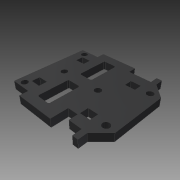
# Autodesk Inventor part: x_motor_middle
Saved by Autodesk Inventor 2014 (Build 180170000, 170)
## iProperties
Created: 2013-12-01
Part Number: x_motor_middle
Material: Generic
Document SubType Name: Modeling
Designer: buben
Density: 1 g/cm^3
Appearance: Anodized - Dark Gray
Author: buben
Subject: Laser Cutted
Autodesk Inventor part; units mm, degrees
ref_plane "YZ Plane" through (0, 0, 0) normal (1, 0, 0) x (0, 1, 0)
ref_plane "XZ Plane" through (0, 0, 0) normal (0, 1, 0) x (-1, 0, 0)
ref_plane "XY Plane" through (0, 0, 0) normal (0, 0, 1) x (1, 0, 0)
sketch "Sketch1" plane through (0, 0, 0) normal (0, 0, 1) x (1, 0, 0)
  line L0 (0, 68.5) -> (0, 6.5)
  line L1 (68, 68.5) -> (78, 58.5)
  line L2 (78, 58.5) -> (78, 16.5)
  line L3 (78, 16.5) -> (68, 6.5)
  line L4 (68, 0) -> (68, 6.5)
  line L5 (68, 68.5) -> (68, 75)
  circle A0 centre (71, 57.5) radius 2.75
  circle A1 centre (71, 17.5) radius 2.75
  line L6 (25, 67.5) -> (34, 67.5)
  line L7 (35, 66.5) -> (35, 43.5)
  line L8 (34, 42.5) -> (25, 42.5)
  line L9 (24, 43.5) -> (24, 66.5)
  line L10 (25, 32.5) -> (34, 32.5)
  line L11 (35, 31.5) -> (35, 8.5)
  line L12 (34, 7.5) -> (25, 7.5)
  line L13 (24, 8.5) -> (24, 31.5)
  arc A2 (25, 67.5) -> (24, 66.5) centre (25, 66.5) ccw
  arc A3 (35, 66.5) -> (34, 67.5) centre (34, 66.5) ccw
  arc A4 (34, 42.5) -> (35, 43.5) centre (34, 43.5) ccw
  arc A5 (24, 43.5) -> (25, 42.5) centre (25, 43.5) ccw
  arc A6 (25, 32.5) -> (24, 31.5) centre (25, 31.5) ccw
  arc A7 (24, 8.5) -> (25, 7.5) centre (25, 8.5) ccw
  arc A8 (34, 7.5) -> (35, 8.5) centre (34, 8.5) ccw
  arc A9 (35, 31.5) -> (34, 32.5) centre (34, 31.5) ccw
  line L14 (29.5, 67.5) -> (29.5, 7.5) construction
  circle A10 centre (6, 64.5) radius 5 construction
  circle A11 centre (6, 64.5) radius 2.75
  circle A12 centre (6, 10.5) radius 5 construction
  circle A13 centre (6, 10.5) radius 2.75
  line L15 (0, 64.5) -> (72, 64.5) construction
  line L16 (0, 10.5) -> (72, 10.5) construction
  line L17 (0, 6.5) -> (16, 6.5)
  line L18 (16, 6.5) -> (16, 0)
  line L19 (0, 68.5) -> (16, 68.5)
  line L20 (16, 68.5) -> (16, 75)
  line L21 (46, 75) -> (46, 68.5)
  line L22 (46, 68.5) -> (64, 68.5)
  line L23 (64, 68.5) -> (64, 75)
  line L24 (46, 0) -> (46, 6.5)
  line L25 (46, 6.5) -> (64, 6.5)
  line L26 (64, 6.5) -> (64, 0)
  line L27 (68, 75) -> (64, 75)
  line L28 (46, 75) -> (16, 75)
  line L29 (16, 0) -> (46, 0)
  line L30 (64, 0) -> (68, 0)
  line L31 (8, 60.5) -> (16, 60.5)
  line L32 (16, 60.5) -> (16, 54)
  line L33 (16, 54) -> (8, 54)
  line L34 (8, 54) -> (8, 60.5)
  line L35 (8, 21) -> (16, 21)
  line L36 (16, 21) -> (16, 14.5)
  line L37 (16, 14.5) -> (8, 14.5)
  line L38 (8, 14.5) -> (8, 21)
  line L39 (54, 21) -> (62, 21)
  line L40 (62, 21) -> (62, 14.5)
  line L41 (62, 14.5) -> (54, 14.5)
  line L42 (54, 14.5) -> (54, 21)
  line L43 (54, 60.5) -> (62, 60.5)
  line L44 (62, 60.5) -> (62, 54)
  line L45 (62, 54) -> (54, 54)
  line L46 (54, 54) -> (54, 60.5)
  circle A14 centre (14, 37.5) radius 5 construction
  circle A15 centre (46, 37.5) radius 5 construction
  circle A16 centre (46, 37.5) radius 2.75
  circle A17 centre (14, 37.5) radius 2.75
  point P0 (0, 0)
  point P1 (29.5, 37.5)
  point P2 (0, 37.5)
  dimension "d1" = 45
  dimension "d2" = 10
  dimension "d11" = 5.5
  dimension "d12" = 5.5
  dimension "d13" = 7
  dimension "d14" = 11
  dimension "d15" = 11
  dimension "d18" = 1
  dimension "d19" = 11
  dimension "d20" = 25
  dimension "d21" = 25
  dimension "d24" = 38.5
  dimension "d25" = 5.5
  dimension "d26" = 5.5
  dimension "d27" = 10
  dimension "d28" = 10
  dimension "d32" = 6
  dimension "d34" = 68
  dimension "d35" = 6.5
  dimension "d36" = 6.5
  dimension "d37" = 4
  dimension "d38" = 4
  dimension "d40" = 1
  dimension "d41" = 30
  dimension "d42" = 18
  dimension "d43" = 4
  dimension "d44" = 4
  dimension "d45" = 6.5
  dimension "d46" = 6.5
  dimension "d47" = 8
  dimension "d48" = 8
  dimension "d49" = 4
  dimension "d50" = 4
  dimension "d51" = 8
  dimension "d52" = 6
  dimension "d53" = 10
  dimension "d54" = 5.5
  dimension "d55" = 10
  dimension "d56" = 5.5
  dimension "d57" = 14
  dimension "d58" = 32
  dimension "d67" = 54
  constraints: 94 end point, 25 parallel, 21 perpendicular, 18 centre point, 17 collinear, 16 point on circle, 16 tangent, 8 horizontal, 7 equal radius, 6 horizontal alignment, 6 point on line, 4 coincident, 4 midpoint, 3 vertical alignment
  measures "d1" angle of L1 L5
  measures "d2" distance between parallel lines of L5 L2
  measures "d11" diameter of A0
  measures "d12" diameter of A1
  measures "d13" distance from line of L2 A1.centre
  measures "d14" vertical distance of L3.end A1.centre
  measures "d15" vertical distance of L1.start A0.centre
  measures "d18" radius of A2
  measures "d19" distance between parallel lines of L7 L9
  measures "d20" distance between parallel lines of L8 L6
  measures "d21" distance between parallel lines of L12 L10
  measures "d24" distance between parallel lines of L5 L14
  measures "d25" diameter of A13
  measures "d26" diameter of A11
  measures "d27" diameter of A10
  measures "d28" diameter of A12
  measures "d32" distance from line of L0 A10.centre
  measures "d34" distance between parallel lines of L4 L0
  measures "d35" distance of L17.end L18.end
  measures "d36" distance of L19.end L20.end
  measures "d37" distance between parallel lines of L5 L23
  measures "d38" distance between parallel lines of L4 L26
  measures "d40" distance between parallel lines of L19 L6
  measures "d41" distance of L18.end L24.start
  measures "d42" distance between parallel lines of L26 L24
  measures "d43" distance between parallel lines of L19 L15
  measures "d44" distance between parallel lines of L17 L16
  measures "d45" distance of L33.end L31.start
  measures "d46" distance of L37.end L35.start
  measures "d47" distance of L31.start L31.end
  measures "d48" distance of L43.start L43.end
  measures "d49" distance between parallel lines of L15 L43
  measures "d50" distance between parallel lines of L16 L41
  measures "d51" distance between parallel lines of L0 L34
  measures "d52" distance from line of L3.end L40
  measures "d53" diameter of A14
  measures "d54" diameter of A17
  measures "d55" diameter of A15
  measures "d56" diameter of A16
  measures "d57" distance from line of L0 A14.centre
  measures "d58" distance from line of L2 A15.centre
  measures "d67" distance between parallel lines of L16 L15
extrude "Extrusion1" add sketch "Sketch1" along normal blind 6.5
sketch "Sketch2" plane through (0, 0, 6.5) normal (0, 0, 1) x (1, 0, 0)
  line L0 (46, 6.5) -> (64, 6.5) projected
  line L1 (46, 13) -> (54, 13)
  line L2 (54, 13) -> (54, 6.5)
  line L3 (54, 6.5) -> (46, 6.5)
  line L4 (46, 6.5) -> (46, 13)
  line L5 (46, 0) -> (46, 6.5) projected
  point P0 (0, 0)
  dimension "d61" = 6.5
  dimension "d62" = 8
  constraints: 8 end point, 2 collinear, 2 parallel, 1 horizontal, 1 perpendicular
  measures "d61" distance of L3.end L1.start
  measures "d62" distance of L1.start L1.end
extrude "Extrusion2" cut sketch "Sketch2" against normal through all
body "Solid1"
